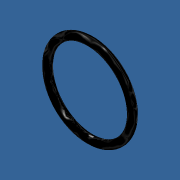
# Autodesk Inventor part: JointTorique
Saved by Autodesk Inventor 2018 (Build 220112000, 112)
## iProperties
Created: 2022-03-22
Part Number: JointTorique
Material: Rubber, Silicone
Document SubType Name: Modeling
Designer: Nathann
Density: 1.25 g/cm^3
Appearance: Rubber - Black
Mass: 0.916023 g
Surface Area: 9.77091 cm^2
Volume: 0.732818 cm^3
Author: Nathann
Autodesk Inventor part; units mm, degrees
ref_plane "YZ Plane" through (0, 0, 0) normal (1, 0, 0) x (0, 1, 0)
ref_plane "XZ Plane" through (0, 0, 0) normal (0, 1, 0) x (-1, 0, 0)
ref_plane "XY Plane" through (0, 0, 0) normal (0, 0, 1) x (1, 0, 0)
sketch "Sketch2" plane through (0, 0, 0) normal (1, 0, 0) x (0, 1, 0)
  circle A0 centre (0, 16.5) radius 1.5
  line L0 (-2.1, 0) -> (2.1, 0) projected
  point P0 (0, 0)
  dimension "d1" = 16.5
  dimension "d2" = 0
  dimension "d3" = 3
  constraints: 1 centre point
  measures "d1" distance of A0.centre point (0, 0)
  measures "d2" horizontal distance of point (0, 0) A0.centre
  measures "d3" diameter of A0
revolve "Revolution1" add sketch "Sketch2" angle 360 about axis through (0, -10, 0) along (0, 1, 0)
equation "\"d1\" = 0.5 * d0"
equation "\"d0\" = 33"
body "Solid1"
